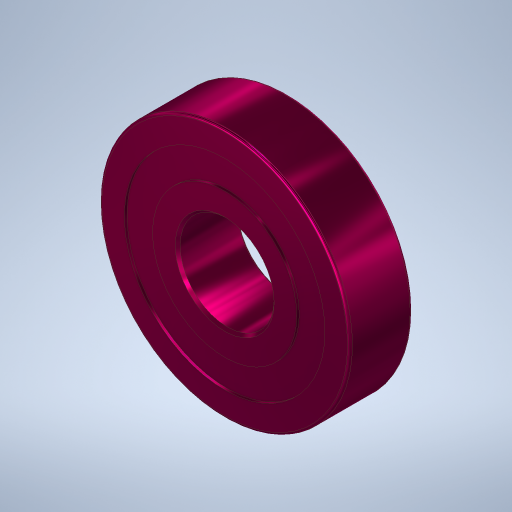
# Autodesk Inventor part: Rear Hub Bearing
Saved by Autodesk Inventor 2023.1 (Build 271208000, 208)
## iProperties
Created: 2019-11-28
Part Number: Rear Hub Bearing
Material: Generic
Document SubType Name: Modeling
Designer: Jopa
Density: 1 g/cm^3
Appearance: Brindle
Author: Jopa
Autodesk Inventor part; units mm, degrees
ref_plane "YZ Plane" through (0, 0, 0) normal (1, 0, 0) x (0, 1, 0)
ref_plane "XZ Plane" through (0, 0, 0) normal (0, 1, 0) x (-1, 0, 0)
sketch "Sketch1" plane through (0, 0, 0) normal (0, 0, 1) x (1, 0, 0)
  circle A0 centre (0, 0) radius 2.3813
  circle A1 centre (0, 0) radius 6.35
  circle A2 centre (0, 0) radius 3.6512
  circle A3 centre (0, 0) radius 5.08
  dimension "d0" = 4.7625
  dimension "d1" = 12.7
  dimension "d2" = 1.27
  dimension "d3" = 1.27
  constraints: 4 centre point, 2 coincident
  measures "d0" diameter of A0
  measures "d1" diameter of A1
  measures "d2" radial gap between concentric circles of A0 A2
  measures "d3" radial gap between concentric circles of A1 A3
extrude "Extrusion1" add sketch "Sketch1" along normal blind 3.175
fillet "Fillet1" radius 0.127 2 edges at (-6.35, 0, 3.175) (-6.35, 0, 0)
chamfer "Chamfer1" distance 0.127 angle 45 2 edges at (-2.3813, 0, 3.175) (-2.3813, 0, 0)
ref_plane "Work Plane1" through (0, 0, 1.5875) normal (0, 0, 1) x (1, 0, 0)
sketch "Sketch2" plane through (0, 0, 1.5875) normal (0, 0, 1) x (1, 0, 0)
  circle A0 centre (0, 0) radius 2.3813 projected
  circle A1 centre (0, 0) radius 3.6512 projected
  circle A2 centre (0, 0) radius 6.35 projected
  circle A3 centre (0, 0) radius 5.08 projected
extrude "Extrusion2" add sketch "Sketch2" along normal mid plane 2.921 contours A3
body "Solid1"
